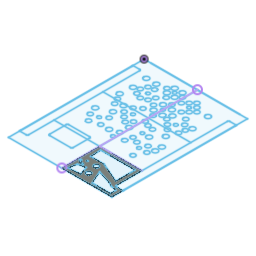
PlayField-ActualSizeHoles v5 (Autodesk Fusion 360 design; units mm, degrees)
Autodesk Fusion 360 part; units mm, degrees
sketch "Sketch2" plane through (0, 0, 0) normal (0, 1, 0) x (1, 0, 0)
  line L0 (0, 0) -> (590.55, 0)
  line L1 (590.55, 0) -> (590.55, -774.7)
  line L2 (590.55, -774.7) -> (0, -774.7)
  line L3 (0, -774.7) -> (0, 0)
  circle A0 centre (101.6, -88.9) radius 14.2875
  circle A1 centre (158.75, -88.9) radius 14.2875
  circle A2 centre (231.775, -57.15) radius 14.2875
  circle A3 centre (276.225, -57.15) radius 14.2875
  circle A4 centre (231.775, -101.6) radius 14.2875
  circle A5 centre (276.225, -101.6) radius 14.2875
  circle A6 centre (466.725, -101.6) radius 14.2875
  circle A7 centre (107.95, -171.45) radius 14.2875
  circle A8 centre (101.6, -241.3) radius 14.2875
  circle A9 centre (279.4, -171.45) radius 14.2875
  circle A10 centre (330.2, -171.45) radius 14.2875
  circle A11 centre (279.4, -225.425) radius 14.2875
  circle A12 centre (330.2, -225.425) radius 14.2875
  circle A13 centre (361.95, -200.025) radius 14.2875
  circle A14 centre (482.6, -206.375) radius 14.2875
  circle A15 centre (101.6, -381) radius 14.2875
  circle A16 centre (295.275, -381) radius 14.2875
  circle A17 centre (485.775, -384.175) radius 14.2875
  circle A18 centre (171.45, -349.25) radius 14.2875
  circle A19 centre (171.45, -288.925) radius 14.2875
  circle A20 centre (444.5, -320.675) radius 14.2875
  circle A21 centre (485.775, -422.275) radius 14.2875
  circle A22 centre (247.65, -447.675) radius 14.2875
  circle A23 centre (444.5, -508) radius 12.7
  circle A24 centre (292.1, -469.9) radius 9.525
  circle A25 centre (425.45, -454.025) radius 9.525
  circle A26 centre (158.75, -415.925) radius 9.525
  circle A27 centre (361.95, -371.475) radius 9.525
  circle A28 centre (241.3, -304.8) radius 9.525
  circle A29 centre (415.925, -234.95) radius 9.525
  circle A30 centre (304.8, -196.85) radius 9.525
  circle A31 centre (180.975, -158.75) radius 9.525
  circle A32 centre (368.3, -111.125) radius 9.525
  circle A33 centre (254, -79.375) radius 9.525
  circle A34 centre (469.9, -454.025) radius 12.7
  circle A35 centre (209.55, -79.375) radius 12.7
  circle A36 centre (298.45, -79.375) radius 12.7
  circle A37 centre (254, -127) radius 12.7
  circle A38 centre (180.975, -120.65) radius 12.7
  circle A39 centre (149.225, -127) radius 12.7
  circle A40 centre (136.525, -158.75) radius 12.7
  circle A41 centre (149.225, -190.5) radius 12.7
  circle A42 centre (180.975, -203.2) radius 12.7
  circle A43 centre (212.725, -190.5) radius 12.7
  circle A44 centre (225.425, -158.75) radius 12.7
  circle A45 centre (304.8, -146.05) radius 12.7
  circle A46 centre (254, -200.025) radius 12.7
  circle A47 centre (323.85, -111.125) radius 12.7
  circle A48 centre (346.075, -88.9) radius 12.7
  circle A49 centre (368.3, -66.675) radius 12.7
  circle A50 centre (390.525, -88.9) radius 12.7
  circle A51 centre (412.75, -111.125) radius 12.7
  circle A52 centre (390.525, -133.35) radius 12.7
  circle A53 centre (368.3, -155.575) radius 12.7
  circle A54 centre (415.925, -177.8) radius 12.7
  circle A55 centre (361.95, -231.775) radius 12.7
  circle A56 centre (441.325, -209.55) radius 12.7
  circle A57 centre (469.9, -234.95) radius 12.7
  circle A58 centre (463.55, -266.7) radius 12.7
  circle A59 centre (241.3, -247.65) radius 12.7
  circle A60 centre (304.8, -254) radius 12.7
  circle A61 centre (120.65, -273.05) radius 12.7
  circle A62 centre (136.525, -304.8) radius 12.7
  circle A63 centre (209.55, -273.05) radius 12.7
  circle A64 centre (203.2, -317.5) radius 12.7
  circle A65 centre (228.6, -342.9) radius 12.7
  circle A66 centre (257.175, -365.125) radius 12.7
  circle A67 centre (279.4, -339.725) radius 12.7
  circle A68 centre (190.5, -390.525) radius 12.7
  circle A69 centre (311.15, -304.8) radius 12.7
  circle A70 centre (339.725, -317.5) radius 12.7
  circle A71 centre (371.475, -323.85) radius 12.7
  circle A72 centre (390.525, -257.175) radius 12.7
  circle A73 centre (415.925, -282.575) radius 12.7
  circle A74 centre (441.325, -419.1) radius 12.7
  circle A75 centre (390.525, -431.8) radius 12.7
  circle A76 centre (355.6, -419.1) radius 12.7
  circle A77 centre (346.075, -457.2) radius 12.7
  circle A78 centre (292.1, -431.8) radius 12.7
  circle A79 centre (200.025, -447.675) radius 12.7
  circle A80 centre (146.05, -463.55) radius 12.7
  circle A81 centre (117.475, -425.45) radius 12.7
  circle A82 centre (400.05, -371.475) radius 14.2875
  circle A83 centre (393.7, -666.75) radius 12.7
  circle A84 centre (406.4, -723.9) radius 12.7
  line L4 (228.6, -539.75) -> (107.95, -539.75)
  spline S0 degree 3 poles (107.95, -539.75) (104.443, -539.75) (101.6, -542.593) (101.6, -546.1) knots 0 0 0 0 1 1 1 1
  line L5 (101.6, -546.1) -> (101.6, -641.35)
  spline S1 degree 3 poles (101.6, -641.35) (101.6, -644.857) (104.443, -647.7) (107.95, -647.7) knots 0 0 0 0 1 1 1 1
  line L6 (107.95, -647.7) -> (228.6, -647.7)
  spline S2 degree 3 poles (228.6, -647.7) (232.107, -647.7) (234.95, -644.857) (234.95, -641.35) knots 0 0 0 0 1 1 1 1
  line L7 (234.95, -641.35) -> (234.95, -546.1)
  spline S3 degree 3 poles (234.95, -546.1) (234.95, -542.593) (232.107, -539.75) (228.6, -539.75) knots 0 0 0 0 1 1 1 1
  circle A85 centre (342.9, -666.75) radius 3.175
  spline S4 degree 3 poles (342.9, -692.15) (333.503, -692.15) (325.3042, -687.0428) (320.9106, -679.4571) knots 0 0 0 0 1 1 1 1
  line L8 (320.9106, -679.4571) -> (320.9099, -679.4578)
  spline S5 degree 3 poles (320.9099, -679.4578) (320.3614, -678.5074) (319.3369, -677.865) (318.1604, -677.865) knots 0 0 0 0 1 1 1 1
  spline S6 degree 3 poles (318.1604, -677.865) (316.4064, -677.865) (314.9854, -679.2863) (314.9854, -681.04) knots 0 0 0 0 1 1 1 1
  spline S7 degree 3 poles (314.9854, -681.04) (314.9854, -681.6206) (315.1434, -682.1622) (315.4154, -682.6303) knots 0 0 0 0 1 1 1 1
  line L9 (315.4154, -682.6303) -> (315.4055, -682.637)
  spline S8 degree 3 poles (315.4055, -682.637) (320.8965, -692.1196) (331.1528, -698.5) (342.9, -698.5) knots 0 0 0 0 1 1 1 1
  spline S9 degree 3 poles (342.9, -698.5) (344.6533, -698.5) (346.075, -697.0786) (346.075, -695.325) knots 0 0 0 0 1 1 1 1
  spline S10 degree 3 poles (346.075, -695.325) (346.075, -693.5714) (344.6533, -692.15) (342.9, -692.15) knots 0 0 0 0 1 1 1 1
  line L10 (38.1, -63.5) -> (0, -63.5)
  line L11 (0, -63.5) -> (0, -69.85)
  line L12 (0, -69.85) -> (0, -704.85)
  line L13 (0, -704.85) -> (0, -711.2)
  line L14 (0, -711.2) -> (38.1, -711.2)
  spline S11 degree 3 poles (38.1, -711.2) (41.607, -711.2) (44.45, -708.357) (44.45, -704.85) knots 0 0 0 0 1 1 1 1
  line L15 (44.45, -704.85) -> (44.45, -69.85)
  spline S12 degree 3 poles (44.45, -69.85) (44.45, -66.343) (41.607, -63.5) (38.1, -63.5) knots 0 0 0 0 1 1 1 1
  line L16 (552.45, -711.2) -> (590.55, -711.2)
  line L17 (590.55, -711.2) -> (590.55, -704.85)
  line L18 (590.55, -704.85) -> (590.55, -69.85)
  line L19 (590.55, -69.85) -> (590.55, -63.5)
  line L20 (590.55, -63.5) -> (552.45, -63.5)
  spline S13 degree 3 poles (552.45, -63.5) (548.943, -63.5) (546.1, -66.343) (546.1, -69.85) knots 0 0 0 0 1 1 1 1
  line L21 (546.1, -69.85) -> (546.1, -704.85)
  spline S14 degree 3 poles (546.1, -704.85) (546.1, -708.357) (548.943, -711.2) (552.45, -711.2) knots 0 0 0 0 1 1 1 1
  line L22 (44.45, -279.4) -> (546.1, -279.4)
  line L23 (546.1, 0) -> (40.4661, 0)
  line L24 (304.8, 0) -> (304.8, -774.7)
  line L25 (44.45, -558.8) -> (546.1, -558.8)
  point P0 (117.475, -88.9)
  point P1 (174.625, -88.9)
  point P2 (247.65, -57.15)
  point P3 (292.1, -57.15)
  point P4 (247.65, -101.6)
  point P5 (292.1, -101.6)
  point P6 (482.6, -101.6)
  point P7 (123.825, -171.45)
  point P8 (117.475, -241.3)
  point P9 (295.275, -171.45)
  point P10 (346.075, -171.45)
  point P11 (295.275, -225.425)
  point P12 (346.075, -225.425)
  point P13 (377.825, -200.025)
  point P14 (498.475, -206.375)
  point P15 (117.475, -381)
  point P16 (311.15, -381)
  point P17 (501.65, -384.175)
  point P18 (187.325, -349.25)
  point P19 (187.325, -288.925)
  point P20 (460.375, -320.675)
  point P21 (501.65, -422.275)
  point P22 (263.525, -447.675)
  point P23 (458.7875, -508)
  point P24 (303.2125, -469.9)
  point P25 (436.5625, -454.025)
  point P26 (169.8625, -415.925)
  point P27 (373.0625, -371.475)
  point P28 (252.4125, -304.8)
  point P29 (427.0375, -234.95)
  point P30 (315.9125, -196.85)
  point P31 (192.0875, -158.75)
  point P32 (379.4125, -111.125)
  point P33 (265.1125, -79.375)
  point P34 (484.1875, -454.025)
  point P35 (223.8375, -79.375)
  point P36 (312.7375, -79.375)
  point P37 (268.2875, -127)
  point P38 (195.2625, -120.65)
  point P39 (163.5125, -127)
  point P40 (150.8125, -158.75)
  point P41 (163.5125, -190.5)
  point P42 (195.2625, -203.2)
  point P43 (227.0125, -190.5)
  point P44 (239.7125, -158.75)
  point P45 (319.0875, -146.05)
  point P46 (268.2875, -200.025)
  point P47 (338.1375, -111.125)
  point P48 (360.3625, -88.9)
  point P49 (382.5875, -66.675)
  point P50 (404.8125, -88.9)
  point P51 (427.0375, -111.125)
  point P52 (404.8125, -133.35)
  point P53 (382.5875, -155.575)
  point P54 (430.2125, -177.8)
  point P55 (376.2375, -231.775)
  point P56 (455.6125, -209.55)
  point P57 (484.1875, -234.95)
  point P58 (477.8375, -266.7)
  point P59 (255.5875, -247.65)
  point P60 (319.0875, -254)
  point P61 (134.9375, -273.05)
  point P62 (150.8125, -304.8)
  point P63 (223.8375, -273.05)
  point P64 (217.4875, -317.5)
  point P65 (242.8875, -342.9)
  point P66 (271.4625, -365.125)
  point P67 (293.6875, -339.725)
  point P68 (204.7875, -390.525)
  point P69 (325.4375, -304.8)
  point P70 (354.0125, -317.5)
  point P71 (385.7625, -323.85)
  point P72 (404.8125, -257.175)
  point P73 (430.2125, -282.575)
  point P74 (455.6125, -419.1)
  point P75 (404.8125, -431.8)
  point P76 (369.8875, -419.1)
  point P77 (360.3625, -457.2)
  point P78 (306.3875, -431.8)
  point P79 (214.3125, -447.675)
  point P80 (160.3375, -463.55)
  point P81 (131.7625, -425.45)
  point P82 (415.925, -371.475)
  point P83 (406.4, -666.75)
  point P84 (417.5125, -723.9)
  point P85 (346.075, -666.75)
  dimension "d6" = 590.55
  dimension "d127" = 279.4
  dimension "d128" = 279.4
  constraint coincident L15 L22.start
  constraint coincident L21 L22.end
  constraint coincident L0 L23.start
  constraint coincident L0 L23.end
  constraint coincident L23 L24.start
  constraint coincident L0 L24.start
  constraint coincident L2 L24.end
  constraint perpendicular L2 L24
  constraint coincident L15 L25.start
  constraint coincident L21 L25.end
  constraint perpendicular L21 L25
  measures "d6" distance of L1 L3
  measures "d127" distance of L22 L23
  measures "d128" distance of L22 L25
extrude "Extrude14" add sketch "Sketch2" along normal blind 1.016 contours L1 L2 L16 L21 S14 L24 L25
sketch "Sketch7" plane through (0, 1.016, 0) normal (0, 1, 0) x (-1, 0, 0)
  circle A0 centre (-406.4, 723.9) radius 12.7
  circle A1 centre (-342.9, 666.75) radius 3.175
  spline S0 degree 3 poles (-342.9, 692.15) (-344.6533, 692.15) (-346.075, 693.5714) (-346.075, 695.325) knots -1 -1 -1 -1 0 0 0 0
  spline S1 degree 3 poles (-346.075, 695.325) (-346.075, 697.0786) (-344.6533, 698.5) (-342.9, 698.5) knots -1 -1 -1 -1 0 0 0 0
  spline S2 degree 3 poles (-342.9, 698.5) (-331.1528, 698.5) (-320.8965, 692.1196) (-315.4055, 682.637) knots -1 -1 -1 -1 0 0 0 0
  line L0 (-315.4055, 682.637) -> (-315.4154, 682.6303)
  spline S3 degree 3 poles (-315.4154, 682.6303) (-315.1434, 682.1622) (-314.9854, 681.6206) (-314.9854, 681.04) knots -1 -1 -1 -1 0 0 0 0
  spline S4 degree 3 poles (-314.9854, 681.04) (-314.9854, 679.2863) (-316.4064, 677.865) (-318.1604, 677.865) knots -1 -1 -1 -1 0 0 0 0
  spline S5 degree 3 poles (-318.1604, 677.865) (-319.3369, 677.865) (-320.3614, 678.5074) (-320.9099, 679.4578) knots -1 -1 -1 -1 0 0 0 0
  line L1 (-320.9099, 679.4578) -> (-320.9106, 679.4571)
  spline S6 degree 3 poles (-320.9106, 679.4571) (-325.3042, 687.0428) (-333.503, 692.15) (-342.9, 692.15) knots -1 -1 -1 -1 0 0 0 0
  circle A2 centre (-393.7, 666.75) radius 12.7
  line L2 (-304.8, 558.8) -> (-304.8, 774.7)
  line L3 (-304.8, 774.7) -> (-590.55, 774.7)
  line L4 (-590.55, 774.7) -> (-590.55, 711.2)
  line L5 (-590.55, 711.2) -> (-552.45, 711.2)
  spline S7 degree 3 poles (-552.45, 711.2) (-548.943, 711.2) (-546.1, 708.357) (-546.1, 704.85) knots -1 -1 -1 -1 0 0 0 0
  line L6 (-546.1, 704.85) -> (-546.1, 558.8)
  line L7 (-304.8, 0) -> (-304.8, 774.7)
  line L8 (-326.9971, 575.4589) -> (-523.6495, 575.4589)
  line L9 (-523.6495, 575.4589) -> (-523.6495, 685.8)
  line L10 (-523.6495, 685.8) -> (-406.4, 635)
  line L11 (-406.4, 635) -> (-330.2, 635)
  line L12 (-330.2, 635) -> (-326.9971, 575.4589)
  line L13 (-569.5639, 761.7156) -> (-465.0247, 761.7156)
  line L14 (-465.0247, 761.7156) -> (-431.8, 685.8)
  line L15 (-431.8, 685.8) -> (-517.2943, 713.2022)
  line L16 (-517.2943, 713.2022) -> (-535.7778, 723.7578)
  line L17 (-535.7778, 723.7578) -> (-569.5089, 729.9378)
  line L18 (-569.5089, 729.9378) -> (-569.5639, 761.7156)
  line L19 (-321.6268, 756.6664) -> (-330.2, 711.2)
  line L20 (-330.2, 711.2) -> (-372.1554, 702.7038)
  line L21 (-372.1554, 702.7038) -> (-388.8348, 750.7796)
  line L22 (-388.8348, 750.7796) -> (-321.6268, 756.6664)
  line L23 (-546.1, 558.8) -> (-304.8, 558.8)
  constraint perpendicular L7 L8
  constraint perpendicular L8 L9
  constraint perpendicular L9 L11
  constraint parallel L11 L13
extrude "Extrude15" cut sketch "Sketch7" against normal blind 1.016 contours L8 L9 L10 L11 L12 | L13 L14 L15 L16 L17 L18 | L19 L20 L21 L22
